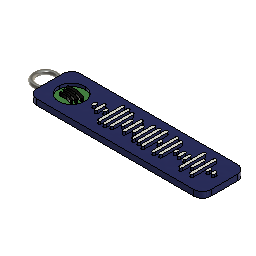
Spotify Code (Autodesk Fusion 360 design; units mm, degrees)
Autodesk Fusion 360 part; units mm, degrees
sketch "Sketch1" plane through (0, 0, 0) normal (0, 0, 1) x (1, 0, 0)
  line L0 (0, 0) -> (105.8333, 0)
  line L1 (105.8333, 0) -> (105.8333, -26.4583)
  line L2 (105.8333, -26.4583) -> (0, -26.4583)
  line L3 (0, -26.4583) -> (0, 0)
  ellipse E0 centre (27.3454, -12.6623) end of major axis (27.973, -13.29) minor radius 0.889 (27.346, -11.774) -> (28.2337, -12.663) cw
  line L4 (28.2337, -12.663) -> (28.2337, -13.7954)
  ellipse E1 centre (27.3453, -13.796) end of major axis (27.973, -14.4237) minor radius 0.889 (28.2337, -13.7954) -> (27.346, -14.6844) cw
  ellipse E2 centre (27.3467, -13.796) end of major axis (27.9744, -14.4237) minor radius 0.889 (27.346, -14.6844) -> (26.4583, -13.7954) cw
  line L5 (26.4583, -13.7954) -> (26.4583, -12.663)
  ellipse E3 centre (27.3467, -12.6623) end of major axis (27.9744, -13.29) minor radius 0.889 (26.4583, -12.663) -> (27.346, -11.774) cw
  ellipse E4 centre (30.6315, -10.8102) end of major axis (31.2592, -11.4379) minor radius 0.889 (30.6321, -9.9219) -> (31.5198, -10.8109) cw
  line L6 (31.5198, -10.8109) -> (31.5198, -15.6475)
  ellipse E5 centre (30.6315, -15.6481) end of major axis (31.2592, -16.2758) minor radius 0.889 (31.5198, -15.6475) -> (30.6321, -16.5365) cw
  ellipse E6 centre (30.6328, -15.6481) end of major axis (31.2605, -16.2758) minor radius 0.889 (30.6321, -16.5365) -> (29.7445, -15.6475) cw
  line L7 (29.7445, -15.6475) -> (29.7445, -10.8109)
  ellipse E7 centre (30.6328, -10.8102) end of major axis (31.2605, -11.4379) minor radius 0.889 (29.7445, -10.8109) -> (30.6321, -9.9219) cw
  ellipse E8 centre (33.9176, -12.6623) end of major axis (34.5453, -13.29) minor radius 0.889 (33.9183, -11.774) -> (34.8059, -12.663) cw
  line L8 (34.8059, -12.663) -> (34.8059, -13.7954)
  ellipse E9 centre (33.9176, -13.796) end of major axis (34.5453, -14.4237) minor radius 0.889 (34.8059, -13.7954) -> (33.9183, -14.6844) cw
  ellipse E10 centre (33.9189, -13.796) end of major axis (34.5466, -14.4237) minor radius 0.889 (33.9183, -14.6844) -> (33.0306, -13.7954) cw
  line L9 (33.0306, -13.7954) -> (33.0306, -12.663)
  ellipse E11 centre (33.9189, -12.6623) end of major axis (34.5466, -13.29) minor radius 0.889 (33.0306, -12.663) -> (33.9183, -11.774) cw
  ellipse E12 centre (37.2064, -6.18) end of major axis (37.8341, -6.8077) minor radius 0.889 (37.207, -5.2917) -> (38.0947, -6.1807) cw
  line L10 (38.0947, -6.1807) -> (38.0947, -20.2777)
  ellipse E13 centre (37.2064, -20.2783) end of major axis (37.8341, -20.906) minor radius 0.889 (38.0947, -20.2777) -> (37.207, -21.1667) cw
  ellipse E14 centre (37.2077, -20.2783) end of major axis (37.8354, -20.906) minor radius 0.889 (37.207, -21.1667) -> (36.3194, -20.2777) cw
  line L11 (36.3194, -20.2777) -> (36.3194, -6.1807)
  ellipse E15 centre (37.2077, -6.18) end of major axis (37.8354, -6.8077) minor radius 0.889 (36.3194, -6.1807) -> (37.207, -5.2917) cw
  ellipse E16 centre (40.4925, -6.18) end of major axis (41.1202, -6.8077) minor radius 0.889 (40.4932, -5.2917) -> (41.3808, -6.1807) cw
  line L12 (41.3808, -6.1807) -> (41.3808, -20.2777)
  ellipse E17 centre (40.4925, -20.2783) end of major axis (41.1202, -20.906) minor radius 0.889 (41.3808, -20.2777) -> (40.4932, -21.1667) cw
  ellipse E18 centre (40.4938, -20.2783) end of major axis (41.1215, -20.906) minor radius 0.889 (40.4932, -21.1667) -> (39.6055, -20.2777) cw
  line L13 (39.6055, -20.2777) -> (39.6055, -6.1807)
  ellipse E19 centre (40.4938, -6.18) end of major axis (41.1215, -6.8077) minor radius 0.889 (39.6055, -6.1807) -> (40.4932, -5.2917) cw
  ellipse E20 centre (43.7786, -7.106) end of major axis (44.4063, -7.7337) minor radius 0.889 (43.7793, -6.2177) -> (44.667, -7.1067) cw
  line L14 (44.667, -7.1067) -> (44.667, -19.3516)
  ellipse E21 centre (43.7786, -19.3523) end of major axis (44.4063, -19.98) minor radius 0.889 (44.667, -19.3516) -> (43.7793, -20.2406) cw
  ellipse E22 centre (43.7799, -19.3523) end of major axis (44.4076, -19.98) minor radius 0.889 (43.7793, -20.2406) -> (42.8916, -19.3516) cw
  line L15 (42.8916, -19.3516) -> (42.8916, -7.1067)
  ellipse E23 centre (43.7799, -7.106) end of major axis (44.4076, -7.7337) minor radius 0.889 (42.8916, -7.1067) -> (43.7793, -6.2177) cw
  ellipse E24 centre (47.0647, -10.8102) end of major axis (47.6924, -11.4379) minor radius 0.889 (47.0654, -9.9219) -> (47.9531, -10.8109) cw
  line L16 (47.9531, -10.8109) -> (47.9531, -15.6475)
  ellipse E25 centre (47.0647, -15.6481) end of major axis (47.6924, -16.2758) minor radius 0.889 (47.9531, -15.6475) -> (47.0654, -16.5365) cw
  ellipse E26 centre (47.0661, -15.6481) end of major axis (47.6937, -16.2758) minor radius 0.889 (47.0654, -16.5365) -> (46.1777, -15.6475) cw
  line L17 (46.1777, -15.6475) -> (46.1777, -10.8109)
  ellipse E27 centre (47.0661, -10.8102) end of major axis (47.6938, -11.4379) minor radius 0.889 (46.1777, -10.8109) -> (47.0654, -9.9219) cw
  ellipse E28 centre (50.3535, -8.0321) end of major axis (50.9812, -8.6598) minor radius 0.889 (50.3542, -7.1438) -> (51.2419, -8.0328) cw
  line L18 (51.2419, -8.0328) -> (51.2419, -18.4256)
  ellipse E29 centre (50.3535, -18.4262) end of major axis (50.9812, -19.0539) minor radius 0.889 (51.2419, -18.4256) -> (50.3542, -19.3146) cw
  ellipse E30 centre (50.3548, -18.4262) end of major axis (50.9825, -19.0539) minor radius 0.889 (50.3542, -19.3146) -> (49.4665, -18.4256) cw
  line L19 (49.4665, -18.4256) -> (49.4665, -8.0328)
  ellipse E31 centre (50.3548, -8.0321) end of major axis (50.9825, -8.6598) minor radius 0.889 (49.4665, -8.0327) -> (50.3542, -7.1438) cw
  ellipse E32 centre (53.6396, -10.8102) end of major axis (54.2673, -11.4379) minor radius 0.889 (53.6403, -9.9219) -> (54.528, -10.8109) cw
  line L20 (54.528, -10.8109) -> (54.528, -15.6475)
  ellipse E33 centre (53.6396, -15.6481) end of major axis (54.2673, -16.2758) minor radius 0.889 (54.528, -15.6475) -> (53.6403, -16.5365) cw
  ellipse E34 centre (53.641, -15.6481) end of major axis (54.2686, -16.2758) minor radius 0.889 (53.6403, -16.5365) -> (52.7526, -15.6475) cw
  line L21 (52.7526, -15.6475) -> (52.7526, -10.8109)
  ellipse E35 centre (53.641, -10.8102) end of major axis (54.2686, -11.4379) minor radius 0.889 (52.7526, -10.8109) -> (53.6403, -9.9219) cw
  ellipse E36 centre (56.9258, -7.106) end of major axis (57.5535, -7.7337) minor radius 0.889 (56.9264, -6.2177) -> (57.8141, -7.1067) cw
  line L22 (57.8141, -7.1067) -> (57.8141, -19.3516)
  ellipse E37 centre (56.9258, -19.3523) end of major axis (57.5534, -19.98) minor radius 0.889 (57.8141, -19.3516) -> (56.9264, -20.2406) cw
  ellipse E38 centre (56.9271, -19.3523) end of major axis (57.5548, -19.98) minor radius 0.889 (56.9264, -20.2406) -> (56.0388, -19.3516) cw
  line L23 (56.0388, -19.3516) -> (56.0388, -7.1067)
  ellipse E39 centre (56.9271, -7.106) end of major axis (57.5548, -7.7337) minor radius 0.889 (56.0388, -7.1067) -> (56.9264, -6.2177) cw
  ellipse E40 centre (60.2119, -7.106) end of major axis (60.8396, -7.7337) minor radius 0.889 (60.2126, -6.2177) -> (61.1002, -7.1067) cw
  line L24 (61.1002, -7.1067) -> (61.1002, -19.3516)
  ellipse E41 centre (60.2119, -19.3523) end of major axis (60.8396, -19.98) minor radius 0.889 (61.1002, -19.3516) -> (60.2126, -20.2406) cw
  ellipse E42 centre (60.2132, -19.3523) end of major axis (60.8409, -19.98) minor radius 0.889 (60.2126, -20.2406) -> (59.3249, -19.3516) cw
  line L25 (59.3249, -19.3516) -> (59.3249, -7.1067)
  ellipse E43 centre (60.2132, -7.106) end of major axis (60.8409, -7.7337) minor radius 0.889 (59.3249, -7.1067) -> (60.2126, -6.2177) cw
  ellipse E44 centre (63.498, -6.18) end of major axis (64.1257, -6.8077) minor radius 0.889 (63.4987, -5.2917) -> (64.3864, -6.1807) cw
  line L26 (64.3864, -6.1807) -> (64.3864, -20.2777)
  ellipse E45 centre (63.498, -20.2783) end of major axis (64.1257, -20.906) minor radius 0.889 (64.3864, -20.2777) -> (63.4987, -21.1667) cw
  ellipse E46 centre (63.4993, -20.2783) end of major axis (64.127, -20.906) minor radius 0.889 (63.4987, -21.1667) -> (62.611, -20.2777) cw
  line L27 (62.611, -20.2777) -> (62.611, -6.1807)
  ellipse E47 centre (63.4993, -6.18) end of major axis (64.127, -6.8077) minor radius 0.889 (62.611, -6.1807) -> (63.4987, -5.2917) cw
  ellipse E48 centre (66.7868, -12.6623) end of major axis (67.4145, -13.29) minor radius 0.889 (66.7874, -11.774) -> (67.6751, -12.663) cw
  line L28 (67.6751, -12.663) -> (67.6751, -13.7954)
  ellipse E49 centre (66.7868, -13.796) end of major axis (67.4145, -14.4237) minor radius 0.889 (67.6751, -13.7954) -> (66.7874, -14.6844) cw
  ellipse E50 centre (66.7881, -13.796) end of major axis (67.4158, -14.4237) minor radius 0.889 (66.7874, -14.6844) -> (65.8998, -13.7954) cw
  line L29 (65.8998, -13.7954) -> (65.8998, -12.663)
  ellipse E51 centre (66.7881, -12.6623) end of major axis (67.4158, -13.29) minor radius 0.889 (65.8998, -12.663) -> (66.7874, -11.774) cw
  ellipse E52 centre (70.0729, -6.18) end of major axis (70.7006, -6.8077) minor radius 0.889 (70.0736, -5.2917) -> (70.9612, -6.1807) cw
  line L30 (70.9613, -6.1807) -> (70.9613, -20.2777)
  ellipse E53 centre (70.0729, -20.2783) end of major axis (70.7006, -20.906) minor radius 0.889 (70.9613, -20.2777) -> (70.0736, -21.1667) cw
  ellipse E54 centre (70.0742, -20.2783) end of major axis (70.7019, -20.906) minor radius 0.889 (70.0736, -21.1667) -> (69.1859, -20.2777) cw
  line L31 (69.1859, -20.2777) -> (69.1859, -6.1807)
  ellipse E55 centre (70.0742, -6.18) end of major axis (70.7019, -6.8077) minor radius 0.889 (69.1859, -6.1807) -> (70.0736, -5.2917) cw
  ellipse E56 centre (73.359, -7.106) end of major axis (73.9867, -7.7337) minor radius 0.889 (73.3597, -6.2177) -> (74.2474, -7.1067) cw
  line L32 (74.2474, -7.1067) -> (74.2474, -19.3516)
  ellipse E57 centre (73.359, -19.3523) end of major axis (73.9867, -19.98) minor radius 0.889 (74.2474, -19.3516) -> (73.3597, -20.2406) cw
  ellipse E58 centre (73.3604, -19.3523) end of major axis (73.988, -19.98) minor radius 0.889 (73.3597, -20.2406) -> (72.472, -19.3516) cw
  line L33 (72.472, -19.3516) -> (72.472, -7.1067)
  ellipse E59 centre (73.3604, -7.106) end of major axis (73.988, -7.7337) minor radius 0.889 (72.472, -7.1067) -> (73.3597, -6.2177) cw
  ellipse E60 centre (76.6452, -12.6623) end of major axis (77.2728, -13.29) minor radius 0.889 (76.6458, -11.774) -> (77.5335, -12.663) cw
  line L34 (77.5335, -12.663) -> (77.5335, -13.7954)
  ellipse E61 centre (76.6452, -13.796) end of major axis (77.2728, -14.4237) minor radius 0.889 (77.5335, -13.7954) -> (76.6458, -14.6844) cw
  ellipse E62 centre (76.6465, -13.796) end of major axis (77.2742, -14.4237) minor radius 0.889 (76.6458, -14.6844) -> (75.7581, -13.7954) cw
  line L35 (75.7581, -13.7954) -> (75.7581, -12.663)
  ellipse E63 centre (76.6465, -12.6623) end of major axis (77.2742, -13.29) minor radius 0.889 (75.7581, -12.663) -> (76.6458, -11.774) cw
  ellipse E64 centre (79.9339, -11.7363) end of major axis (80.5616, -12.3639) minor radius 0.889 (79.9346, -10.8479) -> (80.8223, -11.7369) cw
  line L36 (80.8223, -11.7369) -> (80.8223, -14.7214)
  ellipse E65 centre (79.9339, -14.7221) end of major axis (80.5616, -15.3498) minor radius 0.889 (80.8223, -14.7214) -> (79.9346, -15.6104) cw
  ellipse E66 centre (79.9353, -14.7221) end of major axis (80.5629, -15.3498) minor radius 0.889 (79.9346, -15.6104) -> (79.0469, -14.7214) cw
  line L37 (79.0469, -14.7214) -> (79.0469, -11.7369)
  ellipse E67 centre (79.9353, -11.7363) end of major axis (80.5629, -12.3639) minor radius 0.889 (79.0469, -11.7369) -> (79.9346, -10.8479) cw
  ellipse E68 centre (83.2201, -11.7363) end of major axis (83.8477, -12.3639) minor radius 0.889 (83.2207, -10.8479) -> (84.1084, -11.7369) cw
  line L38 (84.1084, -11.7369) -> (84.1084, -14.7214)
  ellipse E69 centre (83.2201, -14.7221) end of major axis (83.8477, -15.3498) minor radius 0.889 (84.1084, -14.7214) -> (83.2207, -15.6104) cw
  ellipse E70 centre (83.2214, -14.7221) end of major axis (83.8491, -15.3498) minor radius 0.889 (83.2207, -15.6104) -> (82.333, -14.7214) cw
  line L39 (82.333, -14.7214) -> (82.333, -11.7369)
  ellipse E71 centre (83.2214, -11.7363) end of major axis (83.8491, -12.3639) minor radius 0.889 (82.333, -11.7369) -> (83.2207, -10.8479) cw
  ellipse E72 centre (86.5062, -6.18) end of major axis (87.1339, -6.8077) minor radius 0.889 (86.5068, -5.2917) -> (87.3945, -6.1807) cw
  line L40 (87.3945, -6.1807) -> (87.3945, -20.2777)
  ellipse E73 centre (86.5062, -20.2783) end of major axis (87.1339, -20.906) minor radius 0.889 (87.3945, -20.2777) -> (86.5068, -21.1667) cw
  ellipse E74 centre (86.5075, -20.2783) end of major axis (87.1352, -20.906) minor radius 0.889 (86.5068, -21.1667) -> (85.6192, -20.2777) cw
  line L41 (85.6192, -20.2777) -> (85.6192, -6.1807)
  ellipse E75 centre (86.5075, -6.18) end of major axis (87.1352, -6.8077) minor radius 0.889 (85.6192, -6.1807) -> (86.5068, -5.2917) cw
  ellipse E76 centre (89.7923, -9.8842) end of major axis (90.42, -10.5119) minor radius 0.889 (89.793, -8.9958) -> (90.6806, -9.8848) cw
  line L42 (90.6806, -9.8848) -> (90.6806, -16.5735)
  ellipse E77 centre (89.7923, -16.5742) end of major axis (90.42, -17.2018) minor radius 0.889 (90.6806, -16.5735) -> (89.793, -17.4625) cw
  ellipse E78 centre (89.7936, -16.5742) end of major axis (90.4213, -17.2018) minor radius 0.889 (89.793, -17.4625) -> (88.9053, -16.5735) cw
  line L43 (88.9053, -16.5735) -> (88.9053, -9.8848)
  ellipse E79 centre (89.7936, -9.8842) end of major axis (90.4213, -10.5119) minor radius 0.889 (88.9053, -9.8848) -> (89.793, -8.9958) cw
  ellipse E80 centre (93.0784, -6.18) end of major axis (93.7061, -6.8077) minor radius 0.889 (93.0791, -5.2917) -> (93.9668, -6.1807) cw
  line L44 (93.9668, -6.1807) -> (93.9668, -20.2777)
  ellipse E81 centre (93.0784, -20.2783) end of major axis (93.7061, -20.906) minor radius 0.889 (93.9668, -20.2777) -> (93.0791, -21.1667) cw
  ellipse E82 centre (93.0798, -20.2783) end of major axis (93.7074, -20.906) minor radius 0.889 (93.0791, -21.1667) -> (92.1914, -20.2777) cw
  line L45 (92.1914, -20.2777) -> (92.1914, -6.1807)
  ellipse E83 centre (93.0798, -6.18) end of major axis (93.7074, -6.8077) minor radius 0.889 (92.1914, -6.1807) -> (93.0791, -5.2917) cw
  ellipse E84 centre (96.3672, -12.6623) end of major axis (96.9949, -13.29) minor radius 0.889 (96.3679, -11.774) -> (97.2555, -12.663) cw
  line L46 (97.2555, -12.663) -> (97.2555, -13.7954)
  ellipse E85 centre (96.3672, -13.796) end of major axis (96.9949, -14.4237) minor radius 0.889 (97.2555, -13.7954) -> (96.3679, -14.6844) cw
  ellipse E86 centre (96.3685, -13.796) end of major axis (96.9962, -14.4237) minor radius 0.889 (96.3679, -14.6844) -> (95.4802, -13.7954) cw
  line L47 (95.4802, -13.7954) -> (95.4802, -12.663)
  ellipse E87 centre (96.3685, -12.6623) end of major axis (96.9962, -13.29) minor radius 0.889 (95.4802, -12.663) -> (96.3679, -11.774) cw
  ellipse E88 centre (99.6533, -12.6623) end of major axis (100.281, -13.29) minor radius 0.889 (99.654, -11.774) -> (100.5417, -12.663) cw
  line L48 (100.5417, -12.663) -> (100.5417, -13.7954)
  ellipse E89 centre (99.6533, -13.796) end of major axis (100.281, -14.4237) minor radius 0.889 (100.5417, -13.7954) -> (99.654, -14.6844) cw
  ellipse E90 centre (99.6546, -13.796) end of major axis (100.2823, -14.4237) minor radius 0.889 (99.654, -14.6844) -> (98.7663, -13.7954) cw
  line L49 (98.7663, -13.7954) -> (98.7663, -12.663)
  ellipse E91 centre (99.6547, -12.6623) end of major axis (100.2823, -13.29) minor radius 0.889 (98.7663, -12.663) -> (99.654, -11.774) cw
  spline S0 degree 3 poles (13.5439, -5.298) (9.1638, -5.1242) (5.4719, -8.5341) (5.298, -12.9142) knots 0 0 0 0 1 1 1 1
  spline S1 degree 3 poles (5.298, -12.9142) (5.1242, -17.2949) (8.5342, -20.9865) (12.9144, -21.1603) knots 0 0 0 0 1 1 1 1
  spline S2 degree 3 poles (12.9144, -21.1603) (17.2948, -21.3341) (20.9864, -17.9244) (21.1603, -13.5438) knots 0 0 0 0 1 1 1 1
  spline S3 degree 3 poles (21.1603, -13.5438) (21.3341, -9.1637) (17.9243, -5.4718) (13.5439, -5.298) knots 0 0 0 0 1 1 1 1
  spline S4 degree 3 poles (16.8946, -16.926) (16.7956, -17.0998) (16.6033, -17.1872) (16.4165, -17.1609) knots 0 0 0 0 1 1 1 1
  spline S5 degree 3 poles (16.4165, -17.1609) (16.3589, -17.1529) (16.3019, -17.1339) (16.2482, -17.1034) knots 0 0 0 0 1 1 1 1
  spline S6 degree 3 poles (16.2482, -17.1034) (15.1991, -16.5062) (14.0558, -16.1175) (12.8499, -15.948) knots 0 0 0 0 1 1 1 1
  spline S7 degree 3 poles (12.8499, -15.948) (11.6442, -15.7786) (10.438, -15.837) (9.2649, -16.122) knots 0 0 0 0 1 1 1 1
  spline S8 degree 3 poles (9.2649, -16.122) (9.0105, -16.1837) (8.7543, -16.0276) (8.6925, -15.7733) knots 0 0 0 0 1 1 1 1
  spline S9 degree 3 poles (8.6925, -15.7733) (8.6308, -15.5189) (8.7869, -15.2627) (9.0412, -15.2008) knots 0 0 0 0 1 1 1 1
  spline S10 degree 3 poles (9.0412, -15.2008) (10.3312, -14.8876) (11.657, -14.8232) (12.9819, -15.0094) knots 0 0 0 0 1 1 1 1
  spline S11 degree 3 poles (12.9819, -15.0094) (14.3068, -15.1956) (15.5635, -15.623) (16.7171, -16.2796) knots 0 0 0 0 1 1 1 1
  spline S12 degree 3 poles (16.7171, -16.2796) (16.9446, -16.4091) (17.024, -16.6985) (16.8946, -16.926) knots 0 0 0 0 1 1 1 1
  spline S13 degree 3 poles (17.9377, -14.8423) (17.7758, -15.1415) (17.4019, -15.2531) (17.1027, -15.091) knots 0 0 0 0 1 1 1 1
  spline S14 degree 3 poles (17.1027, -15.091) (15.8749, -14.4269) (14.5459, -13.9909) (13.1526, -13.7951) knots 0 0 0 0 1 1 1 1
  spline S15 degree 3 poles (13.1526, -13.7951) (11.7592, -13.5993) (10.3615, -13.652) (8.9981, -13.952) knots 0 0 0 0 1 1 1 1
  spline S16 degree 3 poles (8.9981, -13.952) (8.9243, -13.9683) (8.8508, -13.9706) (8.7801, -13.9607) knots 0 0 0 0 1 1 1 1
  spline S17 degree 3 poles (8.7801, -13.9607) (8.5325, -13.9258) (8.3209, -13.7413) (8.2641, -13.4828) knots 0 0 0 0 1 1 1 1
  spline S18 degree 3 poles (8.2641, -13.4828) (8.191, -13.1505) (8.401, -12.8218) (8.7334, -12.7487) knots 0 0 0 0 1 1 1 1
  spline S19 degree 3 poles (8.7334, -12.7487) (10.2404, -12.417) (11.785, -12.3586) (13.324, -12.5749) knots 0 0 0 0 1 1 1 1
  spline S20 degree 3 poles (13.324, -12.5749) (14.8632, -12.7912) (16.3317, -13.2732) (17.6889, -14.0073) knots 0 0 0 0 1 1 1 1
  spline S21 degree 3 poles (17.6889, -14.0073) (17.9882, -14.1692) (18.0996, -14.543) (17.9377, -14.8423) knots 0 0 0 0 1 1 1 1
  spline S22 degree 3 poles (19.094, -12.4934) (18.9417, -12.7863) (18.6249, -12.9381) (18.3156, -12.8947) knots 0 0 0 0 1 1 1 1
  spline S23 degree 3 poles (18.3156, -12.8947) (18.2326, -12.883) (18.1501, -12.8572) (18.0714, -12.8164) knots 0 0 0 0 1 1 1 1
  spline S24 degree 3 poles (18.0714, -12.8164) (16.642, -12.0731) (15.1024, -11.5816) (13.4953, -11.3558) knots 0 0 0 0 1 1 1 1
  spline S25 degree 3 poles (13.4953, -11.3558) (11.8884, -11.1299) (10.273, -11.178) (8.694, -11.4984) knots 0 0 0 0 1 1 1 1
  spline S26 degree 3 poles (8.694, -11.4984) (8.2835, -11.5817) (7.8833, -11.3165) (7.8001, -10.9062) knots 0 0 0 0 1 1 1 1
  spline S27 degree 3 poles (7.8001, -10.9062) (7.7168, -10.4958) (7.9819, -10.0955) (8.3923, -10.0122) knots 0 0 0 0 1 1 1 1
  spline S28 degree 3 poles (8.3923, -10.0122) (10.1406, -9.6573) (11.9285, -9.6041) (13.7064, -9.854) knots 0 0 0 0 1 1 1 1
  spline S29 degree 3 poles (13.7064, -9.854) (15.4844, -10.1039) (17.1884, -10.6479) (18.7711, -11.4708) knots 0 0 0 0 1 1 1 1
  spline S30 degree 3 poles (18.7711, -11.4708) (19.1426, -11.6641) (19.2871, -12.1219) (19.094, -12.4934) knots 0 0 0 0 1 1 1 1
sketch "Sketch2" plane through (0, 0, 0) normal (0, 0, 1) x (1, 0, 0)
  line L0 (0, -30) -> (60, -30)
  line L1 (0, -30) -> (60.325, -30)
  line L2 (60.325, -30) -> (60.325, -45.0812)
  line L3 (60.325, -45.0812) -> (0, -45.0812)
  line L4 (0, -45.0812) -> (0, -30)
  ellipse E0 centre (15.5869, -37.2175) end of major axis (15.9446, -37.5753) minor radius 0.5067 (15.5872, -36.7112) -> (16.0932, -37.2179) cw
  line L5 (16.0932, -37.2179) -> (16.0932, -37.8634)
  ellipse E1 centre (15.5868, -37.8637) end of major axis (15.9446, -38.2215) minor radius 0.5067 (16.0932, -37.8634) -> (15.5872, -38.3701) cw
  ellipse E2 centre (15.5876, -37.8637) end of major axis (15.9454, -38.2215) minor radius 0.5067 (15.5872, -38.3701) -> (15.0813, -37.8634) cw
  line L6 (15.0813, -37.8634) -> (15.0813, -37.2179)
  ellipse E3 centre (15.5876, -37.2175) end of major axis (15.9454, -37.5753) minor radius 0.5067 (15.0813, -37.2179) -> (15.5872, -36.7112) cw
  ellipse E4 centre (17.4599, -36.1618) end of major axis (17.8177, -36.5196) minor radius 0.5067 (17.4603, -35.6555) -> (17.9663, -36.1622) cw
  line L7 (17.9663, -36.1622) -> (17.9663, -38.9191)
  ellipse E5 centre (17.4599, -38.9194) end of major axis (17.8177, -39.2772) minor radius 0.5067 (17.9663, -38.9191) -> (17.4603, -39.4258) cw
  ellipse E6 centre (17.4607, -38.9194) end of major axis (17.8185, -39.2772) minor radius 0.5067 (17.4603, -39.4258) -> (16.9543, -38.9191) cw
  line L8 (16.9543, -38.9191) -> (16.9543, -36.1622)
  ellipse E7 centre (17.4607, -36.1618) end of major axis (17.8185, -36.5196) minor radius 0.5067 (16.9543, -36.1622) -> (17.4603, -35.6555) cw
  ellipse E8 centre (19.333, -37.2175) end of major axis (19.6908, -37.5753) minor radius 0.5067 (19.3334, -36.7112) -> (19.8394, -37.2179) cw
  line L9 (19.8394, -37.2179) -> (19.8394, -37.8634)
  ellipse E9 centre (19.333, -37.8637) end of major axis (19.6908, -38.2215) minor radius 0.5067 (19.8394, -37.8634) -> (19.3334, -38.3701) cw
  ellipse E10 centre (19.3338, -37.8637) end of major axis (19.6916, -38.2215) minor radius 0.5067 (19.3334, -38.3701) -> (18.8274, -37.8634) cw
  line L10 (18.8274, -37.8634) -> (18.8274, -37.2179)
  ellipse E11 centre (19.3338, -37.2175) end of major axis (19.6916, -37.5753) minor radius 0.5067 (18.8274, -37.2179) -> (19.3334, -36.7112) cw
  ellipse E12 centre (21.2076, -33.5226) end of major axis (21.5654, -33.8804) minor radius 0.5067 (21.208, -33.0163) -> (21.714, -33.523) cw
  line L11 (21.714, -33.523) -> (21.714, -41.5583)
  ellipse E13 centre (21.2076, -41.5586) end of major axis (21.5654, -41.9164) minor radius 0.5067 (21.714, -41.5583) -> (21.208, -42.065) cw
  ellipse E14 centre (21.2084, -41.5586) end of major axis (21.5662, -41.9164) minor radius 0.5067 (21.208, -42.065) -> (20.702, -41.5583) cw
  line L12 (20.702, -41.5583) -> (20.702, -33.523)
  ellipse E15 centre (21.2084, -33.5226) end of major axis (21.5662, -33.8804) minor radius 0.5067 (20.702, -33.523) -> (21.208, -33.0162) cw
  ellipse E16 centre (23.0807, -33.5226) end of major axis (23.4385, -33.8804) minor radius 0.5067 (23.0811, -33.0162) -> (23.5871, -33.523) cw
  line L13 (23.5871, -33.523) -> (23.5871, -41.5583)
  ellipse E17 centre (23.0807, -41.5586) end of major axis (23.4385, -41.9164) minor radius 0.5067 (23.5871, -41.5583) -> (23.0811, -42.065) cw
  ellipse E18 centre (23.0815, -41.5586) end of major axis (23.4393, -41.9164) minor radius 0.5067 (23.0811, -42.065) -> (22.5751, -41.5583) cw
  line L14 (22.5751, -41.5583) -> (22.5751, -33.523)
  ellipse E19 centre (23.0815, -33.5226) end of major axis (23.4393, -33.8804) minor radius 0.5067 (22.5751, -33.523) -> (23.0811, -33.0162) cw
  ellipse E20 centre (24.9538, -34.0504) end of major axis (25.3116, -34.4082) minor radius 0.5067 (24.9542, -33.5441) -> (25.4602, -34.0508) cw
  line L15 (25.4602, -34.0508) -> (25.4602, -41.0304)
  ellipse E21 centre (24.9538, -41.0308) end of major axis (25.3116, -41.3886) minor radius 0.5067 (25.4602, -41.0304) -> (24.9542, -41.5372) cw
  ellipse E22 centre (24.9546, -41.0308) end of major axis (25.3123, -41.3886) minor radius 0.5067 (24.9542, -41.5372) -> (24.4482, -41.0304) cw
  line L16 (24.4482, -41.0304) -> (24.4482, -34.0508)
  ellipse E23 centre (24.9546, -34.0504) end of major axis (25.3123, -34.4082) minor radius 0.5067 (24.4482, -34.0508) -> (24.9542, -33.5441) cw
  ellipse E24 centre (26.8269, -36.1618) end of major axis (27.1847, -36.5196) minor radius 0.5067 (26.8273, -35.6555) -> (27.3333, -36.1622) cw
  line L17 (27.3333, -36.1622) -> (27.3333, -38.9191)
  ellipse E25 centre (26.8269, -38.9194) end of major axis (27.1847, -39.2772) minor radius 0.5067 (27.3333, -38.9191) -> (26.8273, -39.4258) cw
  ellipse E26 centre (26.8277, -38.9194) end of major axis (27.1854, -39.2772) minor radius 0.5067 (26.8273, -39.4258) -> (26.3213, -38.9191) cw
  line L18 (26.3213, -38.9191) -> (26.3213, -36.1622)
  ellipse E27 centre (26.8277, -36.1618) end of major axis (27.1854, -36.5196) minor radius 0.5067 (26.3213, -36.1622) -> (26.8273, -35.6555) cw
  ellipse E28 centre (28.7015, -34.5783) end of major axis (29.0593, -34.9361) minor radius 0.5067 (28.7019, -34.0719) -> (29.2079, -34.5787) cw
  line L19 (29.2079, -34.5787) -> (29.2079, -40.5026)
  ellipse E29 centre (28.7015, -40.503) end of major axis (29.0593, -40.8607) minor radius 0.5067 (29.2079, -40.5026) -> (28.7019, -41.0093) cw
  ellipse E30 centre (28.7023, -40.503) end of major axis (29.06, -40.8607) minor radius 0.5067 (28.7019, -41.0093) -> (28.1959, -40.5026) cw
  line L20 (28.1959, -40.5026) -> (28.1959, -34.5787)
  ellipse E31 centre (28.7023, -34.5783) end of major axis (29.06, -34.9361) minor radius 0.5067 (28.1959, -34.5787) -> (28.7019, -34.0719) cw
  ellipse E32 centre (30.5746, -36.1618) end of major axis (30.9324, -36.5196) minor radius 0.5067 (30.575, -35.6555) -> (31.0809, -36.1622) cw
  line L21 (31.0809, -36.1622) -> (31.0809, -38.9191)
  ellipse E33 centre (30.5746, -38.9194) end of major axis (30.9324, -39.2772) minor radius 0.5067 (31.0809, -38.9191) -> (30.575, -39.4258) cw
  ellipse E34 centre (30.5753, -38.9194) end of major axis (30.9331, -39.2772) minor radius 0.5067 (30.575, -39.4258) -> (30.069, -38.9191) cw
  line L22 (30.069, -38.9191) -> (30.069, -36.1622)
  ellipse E35 centre (30.5753, -36.1618) end of major axis (30.9331, -36.5196) minor radius 0.5067 (30.069, -36.1622) -> (30.575, -35.6555) cw
  ellipse E36 centre (32.4477, -34.0504) end of major axis (32.8055, -34.4082) minor radius 0.5067 (32.4481, -33.5441) -> (32.954, -34.0508) cw
  line L23 (32.954, -34.0508) -> (32.954, -41.0304)
  ellipse E37 centre (32.4477, -41.0308) end of major axis (32.8055, -41.3886) minor radius 0.5067 (32.954, -41.0304) -> (32.4481, -41.5372) cw
  ellipse E38 centre (32.4484, -41.0308) end of major axis (32.8062, -41.3886) minor radius 0.5067 (32.4481, -41.5372) -> (31.9421, -41.0304) cw
  line L24 (31.9421, -41.0304) -> (31.9421, -34.0508)
  ellipse E39 centre (32.4484, -34.0504) end of major axis (32.8062, -34.4082) minor radius 0.5067 (31.9421, -34.0508) -> (32.4481, -33.5441) cw
  ellipse E40 centre (34.3208, -34.0504) end of major axis (34.6786, -34.4082) minor radius 0.5067 (34.3212, -33.5441) -> (34.8271, -34.0508) cw
  line L25 (34.8271, -34.0508) -> (34.8271, -41.0304)
  ellipse E41 centre (34.3208, -41.0308) end of major axis (34.6786, -41.3886) minor radius 0.5067 (34.8271, -41.0304) -> (34.3212, -41.5372) cw
  ellipse E42 centre (34.3215, -41.0308) end of major axis (34.6793, -41.3886) minor radius 0.5067 (34.3212, -41.5372) -> (33.8152, -41.0304) cw
  line L26 (33.8152, -41.0304) -> (33.8152, -34.0508)
  ellipse E43 centre (34.3215, -34.0504) end of major axis (34.6793, -34.4082) minor radius 0.5067 (33.8152, -34.0508) -> (34.3212, -33.5441) cw
  ellipse E44 centre (36.1939, -33.5226) end of major axis (36.5516, -33.8804) minor radius 0.5067 (36.1942, -33.0163) -> (36.7002, -33.523) cw
  line L27 (36.7002, -33.523) -> (36.7002, -41.5583)
  ellipse E45 centre (36.1939, -41.5586) end of major axis (36.5516, -41.9164) minor radius 0.5067 (36.7002, -41.5583) -> (36.1942, -42.065) cw
  ellipse E46 centre (36.1946, -41.5586) end of major axis (36.5524, -41.9164) minor radius 0.5067 (36.1942, -42.065) -> (35.6883, -41.5583) cw
  line L28 (35.6883, -41.5583) -> (35.6883, -33.523)
  ellipse E47 centre (36.1946, -33.5226) end of major axis (36.5524, -33.8804) minor radius 0.5067 (35.6883, -33.523) -> (36.1942, -33.0162) cw
  ellipse E48 centre (38.0685, -37.2175) end of major axis (38.4262, -37.5753) minor radius 0.5067 (38.0688, -36.7112) -> (38.5748, -37.2179) cw
  line L29 (38.5748, -37.2179) -> (38.5748, -37.8634)
  ellipse E49 centre (38.0685, -37.8637) end of major axis (38.4262, -38.2215) minor radius 0.5067 (38.5748, -37.8634) -> (38.0688, -38.3701) cw
  ellipse E50 centre (38.0692, -37.8637) end of major axis (38.427, -38.2215) minor radius 0.5067 (38.0688, -38.3701) -> (37.5629, -37.8634) cw
  line L30 (37.5629, -37.8634) -> (37.5629, -37.2179)
  ellipse E51 centre (38.0692, -37.2175) end of major axis (38.427, -37.5753) minor radius 0.5067 (37.5629, -37.2179) -> (38.0688, -36.7112) cw
  ellipse E52 centre (39.9416, -33.5226) end of major axis (40.2993, -33.8804) minor radius 0.5067 (39.9419, -33.0163) -> (40.4479, -33.523) cw
  line L31 (40.4479, -33.523) -> (40.4479, -41.5583)
  ellipse E53 centre (39.9416, -41.5586) end of major axis (40.2993, -41.9164) minor radius 0.5067 (40.4479, -41.5583) -> (39.9419, -42.065) cw
  ellipse E54 centre (39.9423, -41.5586) end of major axis (40.3001, -41.9164) minor radius 0.5067 (39.9419, -42.065) -> (39.436, -41.5583) cw
  line L32 (39.436, -41.5583) -> (39.436, -33.523)
  ellipse E55 centre (39.9423, -33.5226) end of major axis (40.3001, -33.8804) minor radius 0.5067 (39.436, -33.523) -> (39.9419, -33.0162) cw
  ellipse E56 centre (41.8147, -34.0504) end of major axis (42.1724, -34.4082) minor radius 0.5067 (41.815, -33.5441) -> (42.321, -34.0508) cw
  line L33 (42.321, -34.0508) -> (42.321, -41.0304)
  ellipse E57 centre (41.8147, -41.0308) end of major axis (42.1724, -41.3886) minor radius 0.5067 (42.321, -41.0304) -> (41.815, -41.5372) cw
  ellipse E58 centre (41.8154, -41.0308) end of major axis (42.1732, -41.3886) minor radius 0.5067 (41.815, -41.5372) -> (41.3091, -41.0304) cw
  line L34 (41.3091, -41.0304) -> (41.3091, -34.0508)
  ellipse E59 centre (41.8154, -34.0504) end of major axis (42.1732, -34.4082) minor radius 0.5067 (41.3091, -34.0508) -> (41.815, -33.5441) cw
  ellipse E60 centre (43.6877, -37.2175) end of major axis (44.0455, -37.5753) minor radius 0.5067 (43.6881, -36.7112) -> (44.1941, -37.2179) cw
  line L35 (44.1941, -37.2179) -> (44.1941, -37.8634)
  ellipse E61 centre (43.6877, -37.8637) end of major axis (44.0455, -38.2215) minor radius 0.5067 (44.1941, -37.8634) -> (43.6881, -38.3701) cw
  ellipse E62 centre (43.6885, -37.8637) end of major axis (44.0463, -38.2215) minor radius 0.5067 (43.6881, -38.3701) -> (43.1821, -37.8634) cw
  line L36 (43.1821, -37.8634) -> (43.1821, -37.2179)
  ellipse E63 centre (43.6885, -37.2175) end of major axis (44.0463, -37.5753) minor radius 0.5067 (43.1821, -37.2179) -> (43.6881, -36.7112) cw
  ellipse E64 centre (45.5623, -36.6897) end of major axis (45.9201, -37.0474) minor radius 0.5067 (45.5627, -36.1833) -> (46.0687, -36.69) cw
  line L37 (46.0687, -36.69) -> (46.0687, -38.3912)
  ellipse E65 centre (45.5623, -38.3916) end of major axis (45.9201, -38.7494) minor radius 0.5067 (46.0687, -38.3912) -> (45.5627, -38.8979) cw
  ellipse E66 centre (45.5631, -38.3916) end of major axis (45.9209, -38.7494) minor radius 0.5067 (45.5627, -38.8979) -> (45.0567, -38.3912) cw
  line L38 (45.0567, -38.3912) -> (45.0567, -36.69)
  ellipse E67 centre (45.5631, -36.6897) end of major axis (45.9209, -37.0474) minor radius 0.5067 (45.0567, -36.69) -> (45.5627, -36.1833) cw
  ellipse E68 centre (47.4354, -36.6897) end of major axis (47.7932, -37.0474) minor radius 0.5067 (47.4358, -36.1833) -> (47.9418, -36.69) cw
  line L39 (47.9418, -36.69) -> (47.9418, -38.3912)
  ellipse E69 centre (47.4354, -38.3916) end of major axis (47.7932, -38.7494) minor radius 0.5067 (47.9418, -38.3912) -> (47.4358, -38.8979) cw
  ellipse E70 centre (47.4362, -38.3916) end of major axis (47.794, -38.7494) minor radius 0.5067 (47.4358, -38.8979) -> (46.9298, -38.3912) cw
  line L40 (46.9298, -38.3912) -> (46.9298, -36.69)
  ellipse E71 centre (47.4362, -36.6897) end of major axis (47.794, -37.0474) minor radius 0.5067 (46.9298, -36.69) -> (47.4358, -36.1833) cw
  ellipse E72 centre (49.3085, -33.5226) end of major axis (49.6663, -33.8804) minor radius 0.5067 (49.3089, -33.0162) -> (49.8149, -33.523) cw
  line L41 (49.8149, -33.523) -> (49.8149, -41.5583)
  ellipse E73 centre (49.3085, -41.5586) end of major axis (49.6663, -41.9164) minor radius 0.5067 (49.8149, -41.5583) -> (49.3089, -42.065) cw
  ellipse E74 centre (49.3093, -41.5586) end of major axis (49.6671, -41.9164) minor radius 0.5067 (49.3089, -42.065) -> (48.8029, -41.5583) cw
  line L42 (48.8029, -41.5583) -> (48.8029, -33.523)
  ellipse E75 centre (49.3093, -33.5226) end of major axis (49.6671, -33.8804) minor radius 0.5067 (48.8029, -33.523) -> (49.3089, -33.0162) cw
  ellipse E76 centre (51.1816, -35.634) end of major axis (51.5394, -35.9918) minor radius 0.5067 (51.182, -35.1276) -> (51.688, -35.6344) cw
  line L43 (51.688, -35.6344) -> (51.688, -39.4469)
  ellipse E77 centre (51.1816, -39.4473) end of major axis (51.5394, -39.8051) minor radius 0.5067 (51.688, -39.4469) -> (51.182, -39.9536) cw
  ellipse E78 centre (51.1824, -39.4473) end of major axis (51.5401, -39.8051) minor radius 0.5067 (51.182, -39.9536) -> (50.676, -39.4469) cw
  line L44 (50.676, -39.4469) -> (50.676, -35.6344)
  ellipse E79 centre (51.1824, -35.634) end of major axis (51.5401, -35.9918) minor radius 0.5067 (50.676, -35.6344) -> (51.182, -35.1276) cw
  ellipse E80 centre (53.0547, -33.5226) end of major axis (53.4125, -33.8804) minor radius 0.5067 (53.0551, -33.0162) -> (53.5611, -33.523) cw
  line L45 (53.5611, -33.523) -> (53.5611, -41.5583)
  ellipse E81 centre (53.0547, -41.5586) end of major axis (53.4125, -41.9164) minor radius 0.5067 (53.5611, -41.5583) -> (53.0551, -42.065) cw
  ellipse E82 centre (53.0555, -41.5586) end of major axis (53.4132, -41.9164) minor radius 0.5067 (53.0551, -42.065) -> (52.5491, -41.5583) cw
  line L46 (52.5491, -41.5583) -> (52.5491, -33.523)
  ellipse E83 centre (53.0555, -33.5226) end of major axis (53.4132, -33.8804) minor radius 0.5067 (52.5491, -33.523) -> (53.0551, -33.0162) cw
  ellipse E84 centre (54.9293, -37.2175) end of major axis (55.2871, -37.5753) minor radius 0.5067 (54.9297, -36.7112) -> (55.4357, -37.2179) cw
  line L47 (55.4357, -37.2179) -> (55.4357, -37.8634)
  ellipse E85 centre (54.9293, -37.8637) end of major axis (55.2871, -38.2215) minor radius 0.5067 (55.4357, -37.8634) -> (54.9297, -38.3701) cw
  ellipse E86 centre (54.9301, -37.8637) end of major axis (55.2878, -38.2215) minor radius 0.5067 (54.9297, -38.3701) -> (54.4237, -37.8634) cw
  line L48 (54.4237, -37.8634) -> (54.4237, -37.2179)
  ellipse E87 centre (54.9301, -37.2175) end of major axis (55.2878, -37.5753) minor radius 0.5067 (54.4237, -37.2179) -> (54.9297, -36.7112) cw
  ellipse E88 centre (56.8024, -37.2175) end of major axis (57.1602, -37.5753) minor radius 0.5067 (56.8028, -36.7112) -> (57.3087, -37.2179) cw
  line L49 (57.3088, -37.2179) -> (57.3088, -37.8634)
  ellipse E89 centre (56.8024, -37.8637) end of major axis (57.1602, -38.2215) minor radius 0.5067 (57.3088, -37.8634) -> (56.8028, -38.3701) cw
  ellipse E90 centre (56.8031, -37.8637) end of major axis (57.1609, -38.2215) minor radius 0.5067 (56.8028, -38.3701) -> (56.2968, -37.8634) cw
  line L50 (56.2968, -37.8634) -> (56.2968, -37.2179)
  ellipse E91 centre (56.8032, -37.2175) end of major axis (57.1609, -37.5753) minor radius 0.5067 (56.2968, -37.2179) -> (56.8028, -36.7112) cw
  spline S0 degree 3 poles (7.72, -33.0199) (5.2233, -32.9208) (3.119, -34.8644) (3.0199, -37.3611) knots 0 0 0 0 1 1 1 1
  spline S1 degree 3 poles (3.0199, -37.3611) (2.9208, -39.8581) (4.8645, -41.9623) (7.3612, -42.0614) knots 0 0 0 0 1 1 1 1
  spline S2 degree 3 poles (7.3612, -42.0614) (9.858, -42.1605) (11.9623, -40.2169) (12.0614, -37.72) knots 0 0 0 0 1 1 1 1
  spline S3 degree 3 poles (12.0614, -37.72) (12.1605, -35.2233) (10.2168, -33.119) (7.72, -33.0199) knots 0 0 0 0 1 1 1 1
  spline S4 degree 3 poles (9.6299, -39.6478) (9.5735, -39.7469) (9.4639, -39.7967) (9.3574, -39.7817) knots 0 0 0 0 1 1 1 1
  spline S5 degree 3 poles (9.3574, -39.7817) (9.3246, -39.7771) (9.2921, -39.7663) (9.2615, -39.7489) knots 0 0 0 0 1 1 1 1
  spline S6 degree 3 poles (9.2615, -39.7489) (8.6635, -39.4085) (8.0118, -39.187) (7.3245, -39.0904) knots 0 0 0 0 1 1 1 1
  spline S7 degree 3 poles (7.3245, -39.0904) (6.6372, -38.9938) (5.9497, -39.0271) (5.281, -39.1895) knots 0 0 0 0 1 1 1 1
  spline S8 degree 3 poles (5.281, -39.1895) (5.136, -39.2247) (4.9899, -39.1357) (4.9547, -38.9908) knots 0 0 0 0 1 1 1 1
  spline S9 degree 3 poles (4.9547, -38.9908) (4.9195, -38.8458) (5.0085, -38.6997) (5.1535, -38.6645) knots 0 0 0 0 1 1 1 1
  spline S10 degree 3 poles (5.1535, -38.6645) (5.8888, -38.4859) (6.6445, -38.4492) (7.3997, -38.5554) knots 0 0 0 0 1 1 1 1
  spline S11 degree 3 poles (7.3997, -38.5554) (8.1549, -38.6615) (8.8712, -38.9051) (9.5288, -39.2794) knots 0 0 0 0 1 1 1 1
  spline S12 degree 3 poles (9.5288, -39.2794) (9.6584, -39.3532) (9.7037, -39.5182) (9.6299, -39.6478) knots 0 0 0 0 1 1 1 1
  spline S13 degree 3 poles (10.2245, -38.4601) (10.1322, -38.6307) (9.9191, -38.6943) (9.7486, -38.6019) knots 0 0 0 0 1 1 1 1
  spline S14 degree 3 poles (9.7486, -38.6019) (9.0487, -38.2234) (8.2912, -37.9748) (7.497, -37.8632) knots 0 0 0 0 1 1 1 1
  spline S15 degree 3 poles (7.497, -37.8632) (6.7028, -37.7516) (5.906, -37.7817) (5.1289, -37.9526) knots 0 0 0 0 1 1 1 1
  spline S16 degree 3 poles (5.1289, -37.9526) (5.0869, -37.9619) (5.0449, -37.9632) (5.0047, -37.9576) knots 0 0 0 0 1 1 1 1
  spline S17 degree 3 poles (5.0047, -37.9576) (4.8635, -37.9377) (4.7429, -37.8325) (4.7105, -37.6852) knots 0 0 0 0 1 1 1 1
  spline S18 degree 3 poles (4.7105, -37.6852) (4.6689, -37.4958) (4.7886, -37.3084) (4.978, -37.2667) knots 0 0 0 0 1 1 1 1
  spline S19 degree 3 poles (4.978, -37.2667) (5.837, -37.0777) (6.7174, -37.0444) (7.5947, -37.1677) knots 0 0 0 0 1 1 1 1
  spline S20 degree 3 poles (7.5947, -37.1677) (8.472, -37.291) (9.3091, -37.5657) (10.0827, -37.9842) knots 0 0 0 0 1 1 1 1
  spline S21 degree 3 poles (10.0827, -37.9842) (10.2533, -38.0764) (10.3168, -38.2895) (10.2245, -38.4601) knots 0 0 0 0 1 1 1 1
  spline S22 degree 3 poles (10.8836, -37.1212) (10.7967, -37.2882) (10.6162, -37.3747) (10.4399, -37.35) knots 0 0 0 0 1 1 1 1
  spline S23 degree 3 poles (10.4399, -37.35) (10.3926, -37.3433) (10.3455, -37.3286) (10.3007, -37.3053) knots 0 0 0 0 1 1 1 1
  spline S24 degree 3 poles (10.3007, -37.3053) (9.4859, -36.8816) (8.6083, -36.6015) (7.6923, -36.4728) knots 0 0 0 0 1 1 1 1
  spline S25 degree 3 poles (7.6923, -36.4728) (6.7764, -36.3441) (5.8556, -36.3714) (4.9556, -36.5541) knots 0 0 0 0 1 1 1 1
  spline S26 degree 3 poles (4.9556, -36.5541) (4.7216, -36.6015) (4.4935, -36.4504) (4.446, -36.2165) knots 0 0 0 0 1 1 1 1
  spline S27 degree 3 poles (4.446, -36.2165) (4.3986, -35.9826) (4.5497, -35.7544) (4.7836, -35.707) knots 0 0 0 0 1 1 1 1
  spline S28 degree 3 poles (4.7836, -35.707) (5.7801, -35.5047) (6.7992, -35.4744) (7.8127, -35.6168) knots 0 0 0 0 1 1 1 1
  spline S29 degree 3 poles (7.8127, -35.6168) (8.8261, -35.7592) (9.7974, -36.0693) (10.6995, -36.5384) knots 0 0 0 0 1 1 1 1
  spline S30 degree 3 poles (10.6995, -36.5384) (10.9113, -36.6485) (10.9937, -36.9095) (10.8836, -37.1212) knots 0 0 0 0 1 1 1 1
  dimension "d1" = 60
  constraint horizontal L0
  measures "d1" distance of L0.start L0.end
sketch "Sketch3" plane through (0, 0, 0) normal (0, 0, 1) x (1, 0, 0)
extrude "Extrude1" add sketch "Sketch2" along normal blind 2 contours L0 L1 L2 L3 L4 | E0 L5 E1 E2 L6 E3 | E4 L7 E5 E6 L8 E7 | E8 L9 E9 E10 L10 E11 | E12 L11 E13 E14 L12 E15 | E16 L13 E17 E18 L14 E19 | E20 L15 E21 E22 L16 E23 | E24 L17 E25 E26 L18 E27 | E28 L19 E29 E30 L20 E31 | E32 L21 E33 E34 L22 E35 | E36 L23 E37 E38 L24 E39 | E40 L25 E41 E42 L26 E43 | E44 L27 E45 E46 L28 E47 | E48 L29 E49 E50 L30 E51 | E52 L31 E53 E54 L32 E55 | E56 L33 E57 E58 L34 E59 | E60 L35 E61 E62 L36 E63 | E64 L37 E65 E66 L38 E67 | E68 L39 E69 E70 L40 E71 | E72 L41 E73 E74 L42 E75 | E76 L43 E77 E78 L44 E79 | E80 L45 E81 E82 L46 E83 | E84 L47 E85 E86 L48 E87 | E88 L49 E89 E90 L50 E91 | S0 S1 S2 S3 | S4 S5 S6 S7 S8 S9 S10 S11 S12 | S13 S14 S15 S16 S17 S18 S19 S20 S21 | S22 S23 S24 S25 S26 S27 S28 S29 S30 makes body 1
move_body "Move1" bodies 1 to x (1, 0, 0) y (0, 1, 0) z (0, 0, 1) at (0, 0, -2)
extrude "Extrude2" cut sketch "Sketch2" against normal blind 1 contours S0 S1 S2 S3 bodies 1
extrude "Extrude3" add sketch "Sketch2" along normal blind 1 contours E0 L5 E1 E2 L6 E3 | E4 L7 E5 E6 L8 E7 | E8 L9 E9 E10 L10 E11 | E12 L11 E13 E14 L12 E15 | E16 L13 E17 E18 L14 E19 | E20 L15 E21 E22 L16 E23 | E24 L17 E25 E26 L18 E27 | E28 L19 E29 E30 L20 E31 | E32 L21 E33 E34 L22 E35 | E36 L23 E37 E38 L24 E39 | E40 L25 E41 E42 L26 E43 | E44 L27 E45 E46 L28 E47 | E48 L29 E49 E50 L30 E51 | E52 L31 E53 E54 L32 E55 | E56 L33 E57 E58 L34 E59 | E60 L35 E61 E62 L36 E63 | E64 L37 E65 E66 L38 E67 | E68 L39 E69 E70 L40 E71 | E72 L41 E73 E74 L42 E75 | E76 L43 E77 E78 L44 E79 | E80 L45 E81 E82 L46 E83 | E84 L47 E85 E86 L48 E87 | E88 L49 E89 E90 L50 E91 bodies 1
fillet "Fillet1" radius 3 4 edges at (0, -30, -1) (0, -45.0812, -1) (60.325, -45.0812, -1) (60.325, -30, -1) on bodies 1
torus "TorusPrimitive1" add centre line diameter 7 section diameter 1.5 placed x (1, 0, 0) y (0, 1, 0) z (0, 0, 1) at (-3, -37, 0) separate body makes body 2
move_body "Move2" bodies 2 to x (1, 0, 0) y (0, 1, 0) z (0, 0, 1) at (1, 0, -1)
